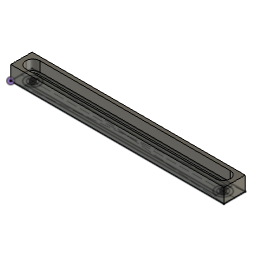
extender v1 (Autodesk Fusion 360 design; units mm, degrees)
Autodesk Fusion 360 part; units mm, degrees
note: some values were not read from the file. Set by a fixed rule: which sketch regions a step uses.
sketch "Sketch1" plane through (0, 0, 0) normal (0, 0, 1) x (1, 0, 0)
  line L0 (0, 0) -> (150, 0)
  line L1 (150, 0) -> (150, 15)
  line L2 (150, 15) -> (0, 15)
  line L3 (0, 15) -> (0, 0)
  line L4 (150, 15) -> (0, 0) construction
  line L5 (0, 15) -> (150, 0) construction
  line L6 (75, 7.5) -> (150, 7.5) construction
  line L7 (75, 7.5) -> (0, 7.5) construction
  circle A0 centre (8, 7.5) radius 5
  circle A1 centre (8, 7.5) radius 3.1375
  circle A2 centre (142, 7.5) radius 5
  circle A3 centre (142, 7.5) radius 3.1375
  line L8 (142, 7.5) -> (142, 15) construction
  line L9 (142, 7.5) -> (142, 0) construction
  line L10 (8, 7.5) -> (8, 15) construction
  line L11 (8, 7.5) -> (8, 0) construction
  line L12 (8, 12.5) -> (142, 12.5)
  line L13 (8, 2.5) -> (142, 2.5)
  line L14 (8, 4.3625) -> (142, 4.3625)
  line L15 (142, 10.6375) -> (8, 10.6375)
  dimension "d1" = 150
  dimension "d2" = 15
  dimension "d3" = 10
  dimension "d4" = 8
  dimension "d5" = 6.275
  dimension "d6" = 10
  dimension "d7" = 8
  dimension "d8" = 6.275
  constraint horizontal L0
  constraint vertical L1
  constraint horizontal L2
  constraint vertical L3
  constraint coincident L0.start L3.end
  constraint midpoint L5 L6.start
  constraint midpoint L1 L6.end
  constraint midpoint L3 L7.end
  constraint coincident L7 A0.centre
  constraint concentric A0 A1
  constraint coincident L6 A2.centre
  constraint concentric A2 A3
  constraint coincident A2.centre A3.centre
  constraint coincident L2 L8.end
  constraint perpendicular L2 L8
  constraint coincident L0 L9.end
  constraint perpendicular L0 L9
  constraint coincident A0.centre A1.centre
  constraint coincident L2 L10.end
  constraint perpendicular L2 L10
  constraint coincident L0 L11.end
  constraint perpendicular L0 L11
  constraint coincident A0 L12.start
  constraint coincident L10 L12.start
  constraint coincident A2 L12.end
  constraint coincident L8 L12.end
  constraint coincident A0 L13.start
  constraint coincident L11 L13.start
  constraint coincident A2 L13.end
  constraint coincident L9 L13.end
  constraint coincident A1 L14.start
  constraint coincident L11 L14.start
  constraint coincident A3 L14.end
  constraint coincident L9 L14.end
  constraint coincident A3 L15.start
  constraint coincident L8 L15.start
  constraint coincident A1 L15.end
  constraint coincident L10 L15.end
  measures "d1" distance of L0.start L0.end
  measures "d2" distance of L0.start L2.end
  measures "d3" diameter of A0
  measures "d4" distance of L3 A0.centre
  measures "d5" diameter of A1
  measures "d6" diameter of A2
  measures "d7" distance of L1 A2.centre
  measures "d8" diameter of A3
extrude "Extrude1" add sketch "Sketch1" along normal blind 10 makes body 1
extrude "Extrude2" add sketch "Sketch1" along normal blind 3 separate body contours A0 A1 L14 L15 | A0 A2 L12 L15 | A0 A2 L13 L14 | A2 A3 L14 L15 picked at (4.0316, 5.6757) picked at (141.753, 3.1392) makes body 2
